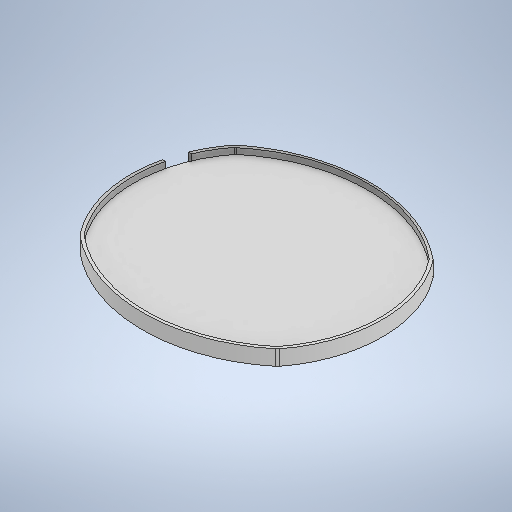
# Autodesk Inventor part: Sonion ring base
Saved by Autodesk Inventor 2025.3 (Build 293356030, 356C)
## iProperties
Created: 2026-07-16
Part Number: Sonion ring base
Material: Generic
Document SubType Name: Modeling
Designer: Samuel Correa Vega
Density: 1 g/cm^3
Appearance: Default
Author: Samuel Correa Vega
Autodesk Inventor part; units mm, degrees
ref_plane "YZ Plane" through (0, 0, 0) normal (1, 0, 0) x (0, 1, 0)
ref_plane "XZ Plane" through (0, 0, 0) normal (0, 1, 0) x (-1, 0, 0)
ref_plane "XY Plane" through (0, 0, 0) normal (0, 0, 1) x (1, 0, 0)
sketch "Sketch11" plane through (0, 0, 0) normal (0, 1, 0) x (-1, 0, 0)
  line L0 (-102.245, 23.8947) -> (-99.7788, 23.8947) projected
  arc A0 (-99.7788, 23.8947) -> (-81.2588, -62.64) centre (0, 0) ccw projected
  arc A1 (-80.0719, -63.8659) -> (80.0719, -63.8659) centre (0, 33.3333) ccw projected
  arc A2 (81.2588, -62.64) -> (81.2588, 62.64) centre (0, 0) ccw projected
  arc A3 (80.0719, 63.8659) -> (-80.0719, 63.8659) centre (0, -33.3333) ccw projected
  arc A4 (-81.2588, 62.64) -> (-94.526, 39.8947) centre (0, 0) ccw projected
  line L1 (-94.526, 39.8947) -> (-97.1257, 39.8947) projected
  arc A5 (-83.1596, 64.1053) -> (-97.1257, 39.8947) centre (0, 0) ccw projected
  arc A6 (81.5979, 65.7183) -> (-81.5979, 65.7183) centre (0, -33.3333) ccw projected
  arc A7 (83.1596, -64.1053) -> (83.1596, 64.1053) centre (0, 0) ccw projected
  arc A8 (-81.5979, -65.7183) -> (81.5979, -65.7183) centre (0, 33.3333) ccw projected
  arc A9 (-102.245, 23.8947) -> (-83.1596, -64.1053) centre (0, 0) ccw projected
  arc A10 (-93.4835, 39.8947) -> (-98.7917, 23.8947) centre (0, 0) ccw projected
  line L2 (-101.282, 23.8947) -> (-98.7917, 23.8947) projected
  arc A11 (-96.1114, 39.8947) -> (-101.282, 23.8947) centre (0, 0) ccw projected
  line L3 (-96.1114, 39.8947) -> (-93.4835, 39.8947) projected
  spline S0 degree 3 poles (366.037, 48.4811) (366.0397, 48.4833) (366.0423, 48.4855) (366.045, 48.4876) (366.0496, 48.4915) (366.0562, 48.4969) (366.154, 48.5774) (366.4584, 48.8288) (367.7198, 49.8494) (368.9391, 50.8224) (371.9742, 53.1167) (373.7879, 54.4353) (378.6033, 57.7188) (381.7908, 59.7316) (388.6525, 63.6242) (392.3319, 65.5095) (403.6984, 70.6488) (411.8775, 73.498) (430.5038, 77.9475) (441.0984, 79.2185) (451.6914, 79.2185) (462.2843, 79.2185) (472.8789, 77.9475) (491.5053, 73.498) (499.6844, 70.6488) (511.0509, 65.5095) (514.7302, 63.6242) (521.5919, 59.7316) (524.7794, 57.7188) (529.5949, 54.4353) (531.4085, 53.1167) (534.4436, 50.8224) (535.663, 49.8494) (536.9243, 48.8288) (537.2288, 48.5774) (537.3265, 48.4969) (537.3332, 48.4915) (537.3378, 48.4876) (537.3404, 48.4855) (537.3431, 48.4833) (537.3457, 48.4811) knots -20.82184 -20.82184 -20.82184 -20.82184 -20.790868 -20.790868 -20.790868 -20.736708 -20.736708 -20.180748 -20.180748 -19.31556 -19.31556 -18.450373 -18.450373 -17.242245 -17.242245 -16.034118 -16.034118 -13.684157 -13.684157 -10.892672 -10.892672 -10.892672 -8.101188 -8.101188 -5.751227 -5.751227 -4.5431 -4.5431 -3.334972 -3.334972 -2.469784 -2.469784 -1.604597 -1.604597 -1.048636 -1.048636 -0.994477 -0.994477 -0.994477 -0.963505 -0.963505 -0.963505 -0.963505
  line L4 (346.379, 7.0643) -> (348.9192, 7.0643)
  arc A12 (354.3296, 23.5443) -> (367.9948, -82.0665) centre (451.6914, -17.5473) ccw
  spline S1 degree 3 poles (367.9948, -82.0665) (368.0665, -82.1595) (368.2141, -82.3423) (368.4475, -82.6062) (368.6926, -82.8593) (368.9488, -83.1012) (369.1267, -83.2546) (369.2173, -83.3292) knots -1 -1 -1 -1 -0.8 -0.6 -0.4 -0.2 0 0 0 0
  arc A13 (369.2173, -83.3292) -> (534.1654, -83.3292) centre (451.6914, 16.786) ccw
  spline S2 degree 3 poles (534.1654, -83.3292) (534.2561, -83.2546) (534.434, -83.1012) (534.6902, -82.8593) (534.9352, -82.6062) (535.1687, -82.3423) (535.3162, -82.1595) (535.3879, -82.0665) knots 0 0 0 0 0.2 0.4 0.6 0.8 1 1 1 1
  arc A14 (535.3879, -82.0665) -> (535.3879, 46.9719) centre (451.6914, -17.5473) ccw
  spline S3 degree 3 poles (535.3879, 46.9719) (535.3162, 47.0649) (535.1687, 47.2476) (534.9352, 47.5115) (534.6902, 47.7647) (534.434, 48.0065) (534.2561, 48.1599) (534.1654, 48.2346) knots -1 -1 -1 -1 -0.8 -0.6 -0.4 -0.2 0 0 0 0
  arc A15 (534.1654, 48.2346) -> (369.2173, 48.2346) centre (451.6914, -51.8807) ccw
  spline S4 degree 3 poles (369.2173, 48.2346) (369.1267, 48.1599) (368.9488, 48.0065) (368.6926, 47.7647) (368.4475, 47.5115) (368.2141, 47.2476) (368.0665, 47.0649) (367.9948, 46.9719) knots 0 0 0 0 0.2 0.4 0.6 0.8 1 1 1 1
  arc A16 (367.9948, 46.9719) -> (354.3296, 23.5443) centre (451.6914, -17.5473) ccw
  line L5 (354.3296, 23.5443) -> (351.6519, 23.5443)
  arc A17 (366.037, 48.4811) -> (351.6519, 23.5443) centre (451.6914, -17.5473) ccw
  spline S5 degree 3 poles (367.6455, 50.1425) (367.3474, 49.8969) (367.0632, 49.6347) (366.5258, 49.0795) (366.2729, 48.7871) (366.037, 48.4811) knots 0 0 0 0 0.112525 0.112525 0.22505 0.22505 0.22505 0.22505
  arc A18 (535.7372, 50.1425) -> (367.6455, 50.1425) centre (451.6914, -51.8807) ccw
  spline S6 degree 3 poles (537.3457, 48.4811) (537.1099, 48.7871) (536.857, 49.0795) (536.3195, 49.6347) (536.0354, 49.8969) (535.7372, 50.1425) knots 0 0 0 0 0.112525 0.112525 0.22505 0.22505 0.22505 0.22505
  arc A19 (537.3457, -83.5757) -> (537.3457, 48.4811) centre (451.6914, -17.5473) ccw
  spline S7 degree 3 poles (535.7372, -85.2372) (536.0354, -84.9915) (536.3195, -84.7293) (536.857, -84.1742) (537.1099, -83.8817) (537.3457, -83.5757) knots 0 0 0 0 0.112525 0.112525 0.22505 0.22505 0.22505 0.22505
  arc A20 (367.6455, -85.2372) -> (535.7372, -85.2372) centre (451.6914, 16.786) ccw
  spline S8 degree 3 poles (366.037, -83.5757) (366.2729, -83.8817) (366.5258, -84.1742) (367.0632, -84.7293) (367.3474, -84.9915) (367.6455, -85.2372) knots 0 0 0 0 0.112525 0.112525 0.22505 0.22505 0.22505 0.22505
  arc A21 (346.379, 7.0643) -> (366.037, -83.5757) centre (451.6914, -17.5473) ccw
  line L6 (347.3709, 7.0643) -> (348.9192, 7.0643)
  arc A22 (352.6966, 23.5443) -> (347.3709, 7.0643) centre (451.6914, -17.5473) ccw
  line L7 (352.6966, 23.5443) -> (354.3296, 23.5443)
  point P0 (354.3296, 23.5443)
  point P1 (348.9192, 7.0643)
  constraints: 23 point on circle, 11 centre point, 8 end point, 2 coincident, 1 horizontal alignment, 30 other
extrude "Extrusion8" add sketch "Sketch11" along normal blind 8 contours A16 S4 A15 S3 A14 S2 A13 S1 A12
sketch "Sketch14" plane through (0, 8, 0) normal (0, 1, 0) x (1, 0, 0)
  line L0 (-557.3026, 42.4254) -> (-554.7623, 42.4254)
  spline S0 degree 3 poles (-535.6868, -46.7054) (-535.6151, -46.7984) (-535.4675, -46.9811) (-535.2341, -47.245) (-534.989, -47.4982) (-534.7328, -47.74) (-534.5549, -47.8934) (-534.4643, -47.9681) knots -1 -1 -1 -1 -0.8 -0.6 -0.4 -0.2 0 0 0 0
  spline S1 degree 3 poles (-537.6446, -48.2146) (-537.4087, -48.5206) (-537.1558, -48.813) (-536.6184, -49.3682) (-536.3342, -49.6304) (-536.036, -49.876) knots 0 0 0 0 0.112525 0.112525 0.22505 0.22505 0.22505 0.22505
  arc A0 (-554.7623, 42.4254) -> (-535.6868, -46.7054) centre (-451.9902, 17.8138) ccw
  arc A1 (-557.3026, 42.4254) -> (-537.6446, -48.2146) centre (-451.9902, 17.8138) ccw
  spline S2 degree 3 poles (-369.5161, -47.9681) (-369.4255, -47.8934) (-369.2476, -47.74) (-368.9914, -47.4982) (-368.7463, -47.245) (-368.5129, -46.9811) (-368.3653, -46.7984) (-368.2937, -46.7054) knots 0 0 0 0 0.2 0.4 0.6 0.8 1 1 1 1
  spline S3 degree 3 poles (-367.9444, -49.876) (-367.6462, -49.6304) (-367.3621, -49.3682) (-366.8246, -48.813) (-366.5717, -48.5206) (-366.3358, -48.2146) knots 0 0 0 0 0.112525 0.112525 0.22505 0.22505 0.22505 0.22505
  arc A2 (-368.2937, -46.7054) -> (-368.2937, 82.333) centre (-451.9902, 17.8138) ccw
  arc A3 (-366.3358, -48.2146) -> (-366.3358, 83.8422) centre (-451.9902, 17.8138) ccw
  spline S4 degree 3 poles (-366.3358, 83.8422) (-366.5717, 84.1482) (-366.8246, 84.4407) (-367.3621, 84.9958) (-367.6462, 85.258) (-367.9444, 85.5037) knots 0 0 0 0 0.112525 0.112525 0.22505 0.22505 0.22505 0.22505
  spline S5 degree 3 poles (-368.2937, 82.333) (-368.3653, 82.426) (-368.5129, 82.6088) (-368.7463, 82.8727) (-368.9914, 83.1258) (-369.2476, 83.3677) (-369.4255, 83.5211) (-369.5161, 83.5957) knots -1 -1 -1 -1 -0.8 -0.6 -0.4 -0.2 0 0 0 0
  spline S6 degree 3 poles (-537.6446, 83.8422) (-537.6419, 83.8444) (-537.6393, 83.8466) (-537.6366, 83.8488) (-537.632, 83.8526) (-537.6253, 83.8581) (-537.5276, 83.9386) (-537.2232, 84.1899) (-535.9618, 85.2106) (-534.7425, 86.1835) (-531.7074, 88.4778) (-529.8937, 89.7964) (-525.0783, 93.08) (-521.8908, 95.0928) (-515.029, 98.9853) (-511.3497, 100.8707) (-499.9832, 106.01) (-491.8041, 108.8591) (-473.1778, 113.3087) (-462.5832, 114.5796) (-451.9902, 114.5796) (-441.3973, 114.5796) (-430.8027, 113.3087) (-412.1763, 108.8591) (-403.9972, 106.01) (-392.6307, 100.8707) (-388.9514, 98.9853) (-382.0897, 95.0928) (-378.9021, 93.08) (-374.0867, 89.7964) (-372.273, 88.4778) (-369.2379, 86.1835) (-368.0186, 85.2106) (-366.7573, 84.1899) (-366.4528, 83.9386) (-366.3551, 83.8581) (-366.3484, 83.8526) (-366.3438, 83.8488) (-366.3411, 83.8466) (-366.3385, 83.8444) (-366.3358, 83.8422) knots -20.82184 -20.82184 -20.82184 -20.82184 -20.790868 -20.790868 -20.790868 -20.736708 -20.736708 -20.180748 -20.180748 -19.31556 -19.31556 -18.450373 -18.450373 -17.242245 -17.242245 -16.034118 -16.034118 -13.684157 -13.684157 -10.892672 -10.892672 -10.892672 -8.101188 -8.101188 -5.751227 -5.751227 -4.5431 -4.5431 -3.334972 -3.334972 -2.469784 -2.469784 -1.604597 -1.604597 -1.048636 -1.048636 -0.994477 -0.994477 -0.994477 -0.963505 -0.963505 -0.963505 -0.963505
  spline S7 degree 3 poles (-534.6619, 82.8298) (-534.7337, 82.8045) (-534.8761, 82.7507) (-535.0858, 82.6604) (-535.2912, 82.5608) (-535.492, 82.4521) (-535.6225, 82.3737) (-535.6868, 82.333) knots 0 0 0 0 0.2 0.4 0.6 0.8 1 1 1 1
  arc A4 (-534.4643, -47.9681) -> (-369.5161, -47.9681) centre (-451.9902, 52.1472) ccw
  arc A5 (-536.036, -49.876) -> (-367.9444, -49.876) centre (-451.9902, 52.1472) ccw
  arc A6 (-367.9444, 85.5037) -> (-536.036, 85.5037) centre (-451.9902, -16.5195) ccw
  arc A7 (-369.5161, 83.5957) -> (-534.6619, 82.8298) centre (-451.6251, -16.8192) ccw
  arc A8 (-535.6868, 82.333) -> (-549.352, 58.9054) centre (-451.9902, 17.8138) ccw
  line L1 (-550.985, 58.9054) -> (-548.2782, 58.9054)
  line L2 (-549.352, 58.9054) -> (-552.0297, 58.9054)
  arc A9 (-548.2782, 58.9054) -> (-553.7457, 42.4254) centre (-451.9902, 17.8138) ccw
  line L3 (-556.3107, 42.4254) -> (-553.7457, 42.4254)
  arc A10 (-550.985, 58.9054) -> (-556.3107, 42.4254) centre (-451.9902, 17.8138) ccw
  arc A11 (-537.6446, 83.8422) -> (-552.0297, 58.9054) centre (-451.9902, 17.8138) ccw
  spline S8 degree 3 poles (-536.036, 85.5037) (-536.3342, 85.258) (-536.6184, 84.9958) (-537.1558, 84.4407) (-537.4087, 84.1482) (-537.6446, 83.8422) knots 0 0 0 0 0.112525 0.112525 0.22505 0.22505 0.22505 0.22505
  line L4 (-349.9359, -7.0643) -> (-348.9192, -7.0643) projected
  line L5 (-349.2823, -7.0643) -> (-349.9359, -7.0643)
  line L6 (-354.3296, -23.5443) -> (-355.4033, -23.5443) projected
  line L7 (-349.9359, -7.0643) -> (-355.4033, -23.5443)
  line L8 (-355.4033, -23.5443) -> (-354.8665, -23.5443)
  point P0 (0, 0)
  point P1 (-537.6446, 83.8422)
  constraints: 25 point on circle, 14 end point, 12 centre point, 1 coincident, 1 collinear, 1 midpoint, 1 point on line, 22 other
extrude "Extrusion11" add sketch "Sketch14" along normal blind 5 and the other way blind 8 contours L0 A0 S0 A4 S2 A2 S5 A7 S7 A8 L1 L2 A11 S6 A3 S3 A5 S1 A1
body "Solid2"
